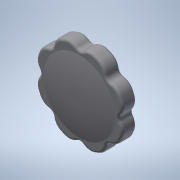
# Autodesk Inventor part: SP34V1 Pomo Cierre
Saved by Autodesk Inventor 2021.2 (Build 252289000, 289)
## iProperties
Created: 2026-08-18
Part Number: SP34V1 Pomo Cierre
Material: Generic
Document SubType Name: Modeling
Designer: nelso
Density: 1 g/cm^3
Appearance: Default
Author: nelso
Autodesk Inventor part; units mm, degrees
ref_plane "YZ Plane" through (0, 0, 0) normal (1, 0, 0) x (0, 1, 0)
ref_plane "XZ Plane" through (0, 0, 0) normal (0, 1, 0) x (-1, 0, 0)
ref_plane "XY Plane" through (0, 0, 0) normal (0, 0, 1) x (1, 0, 0)
sketch "Sketch2" plane through (0, 0, 0) normal (0, 1, 0) x (-1, 0, 0)
  circle A0 centre (0, 0) radius 25
  circle A1 centre (25, 0) radius 3
  circle A2 centre (17.6777, 17.6777) radius 3
  circle A3 centre (0, 25) radius 3
  circle A4 centre (-17.6777, 17.6777) radius 3
  circle A5 centre (-25, 0) radius 3
  circle A6 centre (-17.6777, -17.6777) radius 3
  circle A7 centre (0, -25) radius 3
  circle A8 centre (17.6777, -17.6777) radius 3
  point P0 (-2.9946, 24.82)
  point P1 (2.9946, 24.82)
  point P2 (-15.4329, 19.6679)
  point P3 (-19.6679, 15.4329)
  point P4 (-24.82, 2.9946)
  point P5 (-24.82, -2.9946)
  point P6 (-19.6679, -15.4329)
  point P7 (-15.4329, -19.6679)
  point P8 (2.9946, -24.82)
  point P9 (-2.9946, -24.82)
  point P10 (19.6679, -15.4329)
  point P11 (15.4329, -19.6679)
  point P12 (15.4329, 19.6679)
  point P13 (19.6679, 15.4329)
  point P14 (24.82, 2.9946)
  point P15 (24.82, -2.9946)
  dimension "d11" = 50
  dimension "d12" = 6
  dimension "d15" = 360
  constraints: 8 centre point, 1 coincident, 20 other
  measures "d12" diameter of A1
extrude "Extrusion3" add sketch "Sketch2" along normal mid plane 8 contours A0 A1 | A1 A0 A8 A7 A6 A5 A4 A3 A2 | A2 A0 | A0 A8 | A3 A0 | A0 A7 | A4 A0 | A0 A6 | A5 A0 picked at (24.0535, -0.6751) picked at (17.0479, 16.8839) picked at (16.8839, -17.0479) picked at (-0.116, 23.9934) picked at (0.116, -23.9934) picked at (-16.8963, 17.0326) picked at (-16.8963, -17.0326) picked at (-23.9867, 0)
extrude "Extrusion4" cut sketch "Sketch2" along normal mid plane 8 contours A0 A1 | A2 A0 | A0 A8 | A3 A0 | A0 A7 | A4 A0 | A0 A6 | A5 A0 picked at (24.0535, -0.6751) picked at (17.0479, 16.8839) picked at (16.8839, -17.0479) picked at (-0.116, 23.9934) picked at (0.116, -23.9934) picked at (-16.8963, 17.0326) picked at (-16.8963, -17.0326) picked at (-23.9867, 0)
fillet "Fillet1" radius 7 16 edges at (-19.6679, 0, 15.4329) (-15.4329, 0, 19.6679) (-24.82, 0, 2.9946) (-24.82, 0, -2.9946) (-19.6679, 0, -15.4329) (-15.4329, 0, -19.6679) (-2.9946, 0, -24.82) (2.9946, 0, -24.82) (15.4329, 0, -19.6679) (19.6679, 0, -15.4329) (24.82, 0, -2.9946) (24.82, 0, 2.9946) (19.6679, 0, 15.4329) (15.4329, 0, 19.6679) (-2.9946, 0, 24.82) (2.9946, 0, 24.82)
sketch "Sketch5" plane through (0, 0, 0) normal (1, 0, 0) x (0, 1, 0)
  line L0 (0, 0) -> (6, 0)
  line L1 (4, 1.792) -> (4, -1.792) projected
  line L2 (4, 0) -> (4, 20)
  arc A0 (6, 0) -> (4, 20) centre (-73.9724, 2.1028) ccw
  line L3 (0, 0) -> (0, -26.9215)
  line L4 (0, 0) -> (-6, 0)
  line L5 (-4, 0) -> (-4, 20)
  arc A1 (-4, 20) -> (-6, 0) centre (73.9724, 2.1028) ccw
  point P0 (4, 0)
  dimension "d28" = 6
  dimension "d29" = 20
  dimension "d30" = 80
  constraints: 10 end point, 4 point on circle, 4 symmetric about line, 2 centre point, 2 vertical, 1 horizontal, 1 midpoint, 1 other
  measures "d28" distance of L0.start L0.end
  measures "d29" distance of L2.start L2.end
  measures "d30" radius of A0
revolve "Revolution1" add sketch "Sketch5" angle 360 about axis through (0, 0, 0) along (0, 1, 0)
fillet "Fillet2" radius 2 2 edges at (0, 4, -20) (0, -4, -20)
fillet "Fillet3" radius 1.5 32 edges at (22, 4, 0) (23.9004, 4, 4.9206) (23.9004, 4, -4.9206) (-23.097, 4, 9.5671) (-23.097, 4, -9.5671) (-9.5671, 4, 23.097) (-9.5671, 4, -23.097) (9.5671, 4, 23.097) (9.5671, 4, -23.097) (23.097, 4, 9.5671) (23.097, 4, -9.5671) (13.4207, 4, 20.3795) (20.3795, 4, 13.4208) (15.5563, 4, 15.5563) (-4.9206, 4, 23.9004) (4.9206, 4, 23.9004) (0, 4, 22) (-20.3795, 4, 13.4207) (-13.4207, 4, 20.3795) (-15.5563, 4, 15.5563) (-23.9004, 4, 4.9206) (-23.9004, 4, -4.9206) (-22, 4, 0) (-20.3795, 4, -13.4208) (-13.4208, 4, -20.3795) (-15.5563, 4, -15.5563) (-4.9206, 4, -23.9004) (4.9206, 4, -23.9004) (0, 4, -22) (13.4208, 4, -20.3795) (20.3795, 4, -13.4207) (15.5563, 4, -15.5563)
fillet "Fillet4" radius 1.5 32 edges at (-23.097, -4, 9.5671) (-23.097, -4, -9.5671) (-9.5671, -4, 23.097) (-9.5671, -4, -23.097) (9.5671, -4, 23.097) (9.5671, -4, -23.097) (23.097, -4, 9.5671) (23.097, -4, -9.5671) (23.9004, -4, 4.9206) (23.9004, -4, -4.9206) (22, -4, 0) (13.4208, -4, -20.3795) (20.3795, -4, -13.4207) (15.5563, -4, -15.5563) (-4.9206, -4, -23.9004) (4.9206, -4, -23.9004) (0, -4, -22) (-20.3795, -4, -13.4208) (-13.4208, -4, -20.3795) (-15.5563, -4, -15.5563) (-23.9004, -4, 4.9206) (-23.9004, -4, -4.9206) (-22, -4, 0) (-20.3795, -4, 13.4207) (-13.4207, -4, 20.3795) (-15.5563, -4, 15.5563) (-4.9206, -4, 23.9004) (4.9206, -4, 23.9004) (0, -4, 22) (13.4207, -4, 20.3795) (20.3795, -4, 13.4208) (15.5563, -4, 15.5563)
sketch "Sketch7" plane through (0, 0, 0) normal (0, 1, 0) x (-1, 0, 0)
  circle A0 centre (0, 0) radius 3
  dimension "d35" = 6
  constraints: 1 centre point, 1 coincident
  measures "d35" diameter of A0
extrude "Extrusion5" add sketch "Sketch7" along normal blind 10
body "Solid2"
